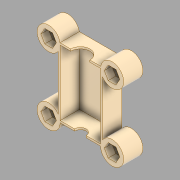
# Autodesk Inventor part: uchwyt_maly_silnik
Saved by Autodesk Inventor 2021 (Build 250183000, 183)
## iProperties
Created: 2022-05-16
Part Number: uchwyt_maly_silnik
Material: PC/ABS Plastic
Document SubType Name: Modeling
Designer: agnpi
Density: 0.357273 g/cm^3
Appearance: Smooth - Off-White
Author: agnpi
Autodesk Inventor part; units mm, degrees
ref_plane "YZ Plane" through (0, 0, 0) normal (1, 0, 0) x (0, 1, 0)
ref_plane "XZ Plane" through (0, 0, 0) normal (0, 1, 0) x (-1, 0, 0)
ref_plane "XY Plane" through (0, 0, 0) normal (0, 0, 1) x (1, 0, 0)
sketch "Sketch1" plane through (0, 0, 0) normal (0, 0, 1) x (1, 0, 0)
  line L0 (-31.5, 0) -> (31.5, 0) projected
  line L1 (0, -33.4) -> (0, 32.4) projected
  line L2 (-10.5, 17) -> (10.5, 17)
  line L3 (10.5, 17) -> (10.5, -17)
  line L4 (10.5, -17) -> (-10.5, -17)
  line L5 (-10.5, -17) -> (-10.5, 17)
  line L6 (-10.5, 17) -> (10.5, -17) construction
  line L7 (10.5, 17) -> (-10.5, -17) construction
  line L8 (-11.5, 18) -> (11.5, 18)
  line L9 (11.5, 18) -> (11.5, -18)
  line L10 (11.5, -18) -> (-11.5, -18)
  line L11 (-11.5, -18) -> (-11.5, 18)
  line L12 (-11.5, 18) -> (11.5, -18) construction
  line L13 (11.5, 18) -> (-11.5, -18) construction
  circle A0 centre (16.5, 17) radius 6
  circle A1 centre (16.5, -18) radius 6
  line L14 (18.5207, 13.5) -> (14.4793, 13.5)
  line L15 (14.4793, 13.5) -> (12.4585, 17)
  line L16 (12.4585, 17) -> (14.4793, 20.5)
  line L17 (14.4793, 20.5) -> (18.5207, 20.5)
  line L18 (18.5207, 20.5) -> (20.5415, 17)
  line L19 (20.5415, 17) -> (18.5207, 13.5)
  line L20 (18.5207, -21.5) -> (14.4793, -21.5)
  line L21 (14.4793, -21.5) -> (12.4585, -18)
  line L22 (12.4585, -18) -> (14.4793, -14.5)
  line L23 (14.4793, -14.5) -> (18.5207, -14.5)
  line L24 (18.5207, -14.5) -> (20.5415, -18)
  line L25 (20.5415, -18) -> (18.5207, -21.5)
  circle A2 centre (-16.5, -18) radius 6
  circle A3 centre (-16.5, 17) radius 6
  point P0 (0, 0)
  point P1 (-11.5, -14.6834)
  point P2 (-10.5, -18)
  point P3 (-10.5839, 18)
  point P4 (-11.5, 13.6834)
  dimension "d0" = 21
  dimension "d1" = 34
  dimension "d2" = 23
  dimension "d3" = 36
  dimension "d13" = 12
  dimension "d14" = 12
  dimension "d15" = 47
  dimension "d16" = 0
  dimension "d18" = 7
  dimension "d19" = 7
  constraints: 48 end point, 6 parallel, 4 centre point, 4 midpoint, 2 coincident, 2 horizontal, 2 perpendicular, 2 symmetric about line, 2 tangent, 28 other
  measures "d0" distance of L3.end L4.end
  measures "d1" distance of L2.end L3.end
  measures "d2" distance of L9.end L10.end
  measures "d3" distance of L8.end L9.end
  measures "d13" diameter of A0
  measures "d14" diameter of A1
  measures "d16" distance from line of L2 A0.centre
  measures "d18" distance between parallel lines of L14 L17
  measures "d19" distance between parallel lines of L20 L23
extrude "Extrusion1" add sketch "Sketch1" along normal blind 10 contours L11 A3 L5 L0 | L0 L5 L4 L1 L10 A2 L11 | A2 L10 L11 | L11 L8 A3 | A3 L8 L1 L2 | L3 A0 L9 L0 | L0 L9 A1 L10 L1 L4 L3 | L1 L8 A0 L2 | A0 L8 L9 | A1 L9 L10 picked at (-11.3172, -16.1332) picked at (-11.3172, 15.4666) picked at (11.3172, 15.4666) picked at (11.3172, -16.1332)
extrude "Extrusion2" add sketch "Sketch1" along normal blind 10 contours A0 L8 L9 | A0 L9 L8 | L14 L15 L16 L17 L18 L19
sketch "Sketch3" plane through (-11.5, -18, 10) normal (0, -1, 0) x (1, 0, 0)
  line L0 (23, 0) -> (0, 0) projected
  arc A0 (8.5, 0) -> (14.5, 0) centre (11.5, 0) ccw
  point P0 (11.5, -10)
  point P1 (14.5, 0)
  dimension "d36" = 3
  dimension "d108" = 6
  constraints: 2 point on circle, 1 centre point, 1 midpoint, 1 point on line
  measures "d36" radius of A0
  measures "d108" distance of A0.end A0.start
extrude "Extrusion6" cut sketch "Sketch3" against normal up to surface (1 mm away)
sketch "Sketch4" plane through (-11.5, 18, 10) normal (0, 1, 0) x (1, 0, 0)
  arc A0 (14.5, 0) -> (8.5, 0) centre (11.5, 0) ccw projected
  line L0 (1, 0) -> (22, 0) projected
  arc A1 (16.5, 0) -> (6.5, 0) centre (11.5, 0) ccw
  point P0 (11.5, 10)
  point P1 (6.5, 0)
  dimension "d39" = 5
  constraints: 2 point on circle, 1 centre point, 1 coincident, 1 point on line
  measures "d39" radius of A1
extrude "Extrusion7" cut sketch "Sketch4" against normal up to surface (1 mm away)
extrude "Extrusion8" add sketch "Sketch1" against normal blind 0.01 contours L5 L2 L1 L0 | L0 L1 L4 L5 | L1 L2 L3 L0 | L0 L3 L4 L1
hole "Hole2" at (16.5, 17, 0) direction (0, 0, 1) diameter 4 end through all
extrude "Extrusion10" add sketch "Sketch1" along normal blind 10 contours L11 L10 A2 picked at (-18.7986, -18.1791)
sketch "Sketch6" plane through (0, 0, 10) normal (0, 0, 1) x (1, 0, 0)
  line L0 (18.5207, 13.5) -> (14.4793, 13.5)
  line L1 (14.4793, 13.5) -> (12.4586, 17)
  line L2 (12.4586, 17) -> (14.4793, 20.5)
  line L3 (14.4793, 20.5) -> (18.5207, 20.5)
  line L4 (18.5207, 20.5) -> (20.5415, 17)
  line L5 (20.5415, 17) -> (18.5207, 13.5)
  line L6 (5, 17) -> (10.5, 17) projected
  point P0 (0, 0)
  point P1 (16.5, 17)
  dimension "d56" = 7
  constraints: 12 end point, 1 parallel, 13 other
  measures "d56" distance between parallel lines of L0 L3
extrude "Extrusion11" cut sketch "Sketch6" against normal blind 4
extrude "Extrusion12" add sketch "Sketch1" along normal blind 10 contours A1 L9 L10 | L10 L9 A1 | L20 L21 L22 L23 L24 L25
hole "Hole3" at (16.5, -18, 0) direction (0, 0, 1) diameter 4 end through all
hole "Hole4" at (-16.5, -18, 0) direction (0, 0, 1) diameter 4 end through all
sketch "Sketch7" plane through (0, 0, 10) normal (0, 0, 1) x (1, 0, 0)
  line L0 (-14.4793, -21.5) -> (-18.5207, -21.5)
  line L1 (-18.5207, -21.5) -> (-20.5415, -18)
  line L2 (-20.5415, -18) -> (-18.5207, -14.5)
  line L3 (-18.5207, -14.5) -> (-14.4793, -14.5)
  line L4 (-14.4793, -14.5) -> (-12.4585, -18)
  line L5 (-12.4585, -18) -> (-14.4793, -21.5)
  line L6 (-10.5, -18) -> (-3, -18) projected
  line L7 (-10.5, 17) -> (-5, 17) projected
  point P0 (0, 0)
  point P1 (-16.5, -18)
  dimension "d75" = 7
  dimension "d78" = 31.5
  dimension "d79" = 19.7894
  constraints: 12 end point, 1 parallel, 13 other
  measures "d75" distance between parallel lines of L0 L3
  measures "d78" distance between parallel lines of L7 L3
  measures "d79" distance from line of point (0, 0) L4
extrude "Extrusion13" add sketch "Sketch1" along normal blind 10 contours A3 L8 L11 picked at (-18.6587, 16.2674)
sketch "Sketch8" plane through (0, 0, 10) normal (0, 0, 1) x (1, 0, 0)
  point P0 (0, 0)
hole "Hole5" at (-16.5, 17, 0) direction (0, 0, 1) diameter 4 end through all
sketch "Sketch9" plane through (0, 0, 10) normal (0, 0, 1) x (1, 0, 0)
  line L0 (-14.4793, 13.5) -> (-18.5207, 13.5)
  line L1 (-18.5207, 13.5) -> (-20.5414, 17)
  line L2 (-20.5414, 17) -> (-18.5207, 20.5)
  line L3 (-18.5207, 20.5) -> (-14.4793, 20.5)
  line L4 (-14.4793, 20.5) -> (-12.4585, 17)
  line L5 (-12.4585, 17) -> (-14.4793, 13.5)
  line L6 (-10.5, 17) -> (-5, 17) projected
  point P0 (0, 0)
  point P1 (-16.5, 17)
  dimension "d89" = 7
  dimension "d90" = 2.2894
  constraints: 12 end point, 1 parallel, 1 point on line, 13 other
  measures "d89" distance between parallel lines of L0 L3
  measures "d90" distance from line of point (0, 0) L4
extrude "Extrusion14" cut sketch "Sketch9" against normal blind 4
extrude "Extrusion15" cut sketch "Sketch7" against normal blind 4
sketch "Sketch10" plane through (0, 0, 10) normal (0, 0, 1) x (1, 0, 0)
  line L0 (18.5207, -21.4318) -> (14.4793, -21.4318)
  line L1 (14.4793, -21.4318) -> (12.4585, -17.9318)
  line L2 (12.4585, -17.9318) -> (14.4793, -14.4318)
  line L3 (14.4793, -14.4318) -> (18.5207, -14.4318)
  line L4 (18.5207, -14.4318) -> (20.5415, -17.9318)
  line L5 (20.5415, -17.9318) -> (18.5207, -21.4318)
  line L6 (3, -18) -> (10.5, -18) projected
  arc A0 (11.5, 13.6834) -> (10.5839, 18) centre (16.5, 17) ccw projected
  point P0 (0, 0)
  point P1 (16.5, -17.9318)
  dimension "d95" = 7
  dimension "d96" = 34.9318
  dimension "d97" = 13.9659
  constraints: 12 end point, 1 parallel, 13 other
  measures "d95" distance between parallel lines of L0 L3
  measures "d96" distance of A0.centre point (16.5, -17.932)
  measures "d97" distance from line of A0.centre L4
extrude "Extrusion16" cut sketch "Sketch10" against normal blind 4
sketch "Sketch11" plane through (0, -18, 10) normal (0, -1, 0) x (1, 0, 0)
  circle A0 centre (0, -6) radius 2
  line L0 (-10.5, -10) -> (10.5, -10) projected
  arc A1 (-3, 0) -> (3, 0) centre (0, 0) ccw projected
  point P0 (0, -10)
  dimension "d100" = 4
  dimension "d101" = 2
  dimension "d109" = 1
  constraints: 1 centre point
  measures "d100" diameter of A0
  measures "d101" distance edge to line of A0 L0
extrude "Extrusion17" cut sketch "Sketch11" against normal blind 0.3
body "Solid1"
